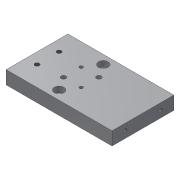
# Autodesk Inventor part: 23-0064 Base plate
Saved by Autodesk Inventor 2022.4 (Build 264492000, 492)
## iProperties
Category: -
Company: Universiteit van Amsterdam
Created: 2023-09-04
Part Number: 23-0064 Base plate
Material: ALMg4,5Mn-5083-(D54S)
Document SubType Name: Modeling
Designer: Ronald Hassing
Density: 2.66 g/cm^3
Appearance: Aluminum - Flat(2)
User Status: Work in Progress
Author: Ronald Hassing
Revision Number: A
Autodesk Inventor part; units mm, degrees
ref_plane "YZ Plane" through (0, 0, 0) normal (1, 0, 0) x (0, 1, 0)
ref_plane "XZ Plane" through (0, 0, 0) normal (0, 1, 0) x (-1, 0, 0)
ref_plane "XY Plane" through (0, 0, 0) normal (0, 0, 1) x (1, 0, 0)
sketch "Sketch1" plane through (0, 0, 0) normal (0, 0, 1) x (1, 0, 0)
  line L0 (0, 49) -> (0, -49) construction
  line L1 (-74, 0) -> (94, 0) construction
  line L2 (-50, -35) -> (70, -35)
  line L3 (70, -35) -> (70, 35)
  line L4 (70, 35) -> (-50, 35)
  line L5 (-50, 35) -> (-50, -35)
  point P0 (0, 0)
  dimension "d4" = 70
  dimension "d49" = 120
  dimension "d50" = 50
  dimension "d51" = 35
  constraints: 8 end point, 2 parallel, 1 horizontal, 1 perpendicular
  measures "d4" distance of L4.end L2.start
  measures "d49" distance of L3.end L4.end
  measures "d50" distance from line of L5 point (0, 0)
  measures "d51" distance between parallel lines of L1 L4
extrude "Extrusion3" add sketch "Sketch1" along normal blind 15
sketch "Sketch2" plane through (0, 0, 15) normal (0, 0, 1) x (1, 0, 0)
  point P0 (0, 0)
  point P1 (0, -25)
  point P2 (0, 25)
  dimension "d15" = 25
  dimension "d16" = 25
  constraints: 2 vertical alignment
  measures "d15" distance of point (0, 25) point (0, 0)
  measures "d16" distance of point (0, -25) point (0, 0)
hole "Hole1" at (0, -25, 15) at (0, 25, 15) direction (0, 0, -1) diameter 6.6 end through all counterbore diameter 11 counterbore depth 6.6 clearance for "Socket Head Cap Screw DIN EN ISO 4762" size "M6" standard "DIN"
sketch "Sketch3" plane through (0, 0, 15) normal (0, 0, 1) x (1, 0, 0)
  point P0 (0, 0)
  point P1 (-37.5, -12.5)
  point P2 (-37.5, 12.5)
  dimension "d24" = 25
  dimension "d25" = 12.5
  dimension "d26" = 37.5
  constraints: 1 vertical alignment
  measures "d24" distance of point (-37.5, 12.5) point (-37.5, -12.5)
  measures "d25" vertical distance of point (-37.5, 12.5) point (0, 0)
  measures "d26" horizontal distance of point (-37.5, 12.5) point (0, 0)
hole "Hole2" at (-37.5, -12.5, 15) at (-37.5, 12.5, 15) direction (0, 0, -1) diameter 4.917 end through all thread size "M6x1" class "6H" standard "ISO Metric profile"
sketch "Sketch4" plane through (0, 0, 0) normal (0, 0, -1) x (-1, 0, 0)
  point P0 (0, 0)
  point P1 (10, -10)
  point P2 (-10, 10)
  dimension "d34" = 10
  dimension "d35" = 10
  dimension "d36" = 10
  dimension "d37" = 10
  measures "d34" horizontal distance of point (-10, 10) point (0, 0)
  measures "d35" horizontal distance of point (10, -10) point (0, 0)
  measures "d36" horizontal distance of point (0, 0) point (-10, 10)
  measures "d37" horizontal distance of point (0, 0) point (10, -10)
hole "Hole3" at (-10, -10, 0) at (10, 10, 0) direction (0, 0, 1) diameter 5.5 end through all counterbore diameter 10 counterbore depth 5.5 clearance for "Socket Head Cap Screw DIN EN ISO 4762" size "M5" standard "DIN"
sketch "Sketch5" plane through (0, 0, 15) normal (0, 0, 1) x (1, 0, 0)
  point P0 (0, 0)
  point P1 (10, -10)
  point P2 (-10, 10)
  dimension "d45" = 10
  dimension "d46" = 10
  dimension "d47" = 10
  dimension "d48" = 10
  measures "d45" horizontal distance of point (10, -10) point (0, 0)
  measures "d46" horizontal distance of point (-10, 10) point (0, 0)
  measures "d47" horizontal distance of point (0, 0) point (10, -10)
  measures "d48" horizontal distance of point (-10, 10) point (0, 0)
hole "Hole4" at (10, -10, 15) at (-10, 10, 15) direction (0, 0, -1) diameter 4 depth 10 tip angle 118
sketch "Sketch6" plane through (70, -35, 0) normal (1, 0, 0) x (0, 0, -1)
  line L0 (0, 0) -> (-15, 0) projected
  line L1 (0, 0) -> (0, 70) projected
  point P0 (0, 35)
  point P1 (-7.5, 15)
  point P2 (-7.5, 55)
  point P3 (-7.5, 0)
  point P4 (0, 35)
  point P5 (0, 35)
  dimension "d59" = 20
  dimension "d60" = 20
  constraints: 3 midpoint, 2 vertical alignment
  measures "d59" vertical distance of point (-7.5, 15) point (0, 35)
  measures "d60" vertical distance of point (-7.5, 55) point (0, 35)
hole "Hole5" at (70, -20, 7.5) at (70, 20, 7.5) direction (-1, 0, 0) diameter 4.134 depth 15 tip angle 118 thread size "M5x0.8" class "6H" standard "ISO Metric profile"
body "Solid3"
